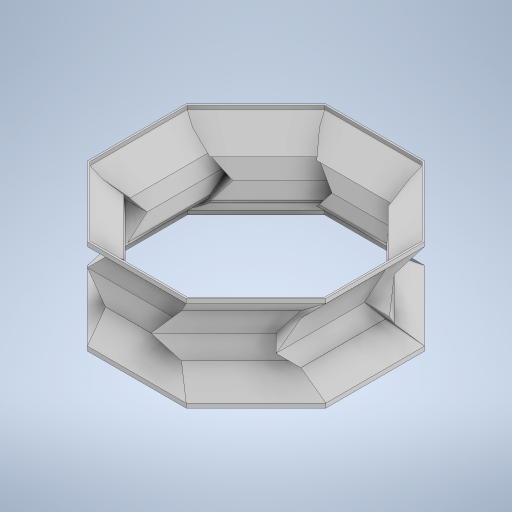
# Autodesk Inventor part: OV-PAM_new_shape
Saved by Autodesk Inventor 2024 (Build 280153000, 153)
## iProperties
Created: 2023-06-16
Part Number: OV-PAM_new_shape
Material: 일반
Document SubType Name: Modeling
Designer: jsw
Density: 1 g/cm^3
Appearance: 기본값
Author: jsw
Autodesk Inventor part; units mm, degrees
sketch "스케치1" plane through (0, 0, 0) normal (0, 1, 0) x (-1, 0, 0)
  line L0 (-32.5919, 13.5) -> (-13.5, 32.5919)
  line L1 (-13.5, 32.5919) -> (13.5, 32.5919)
  line L2 (13.5, 32.5919) -> (32.5919, 13.5)
  line L3 (32.5919, 13.5) -> (32.5919, -13.5)
  line L4 (32.5919, -13.5) -> (13.5, -32.5919)
  line L5 (13.5, -32.5919) -> (-13.5, -32.5919)
  line L6 (-13.5, -32.5919) -> (-32.5919, -13.5)
  line L7 (-32.5919, -13.5) -> (-32.5919, 13.5)
  line L8 (-13.7485, 33.1919) -> (13.7485, 33.1919)
  line L9 (13.7485, 33.1919) -> (33.1919, 13.7485)
  line L10 (33.1919, 13.7485) -> (33.1919, -13.7485)
  line L11 (33.1919, -13.7485) -> (13.7485, -33.1919)
  line L12 (13.7485, -33.1919) -> (-13.7485, -33.1919)
  line L13 (-13.7485, -33.1919) -> (-33.1919, -13.7485)
  line L14 (-33.1919, -13.7485) -> (-33.1919, 13.7485)
  line L15 (-33.1919, 13.7485) -> (-13.7485, 33.1919)
  point P0 (0, 0)
  point P1 (0, 0)
  point P2 (0, 0)
  dimension "d0" = 27
  dimension "d2" = 0.6
  constraints: 32 end point, 2 coincident, 2 horizontal, 34 other
  measures "d0" distance of L0.end L1.end
  measures "d2" distance between parallel lines of L10 L3
extrude "돌출2" add sketch "스케치1" along normal blind 12 contours L0 L1 L2 L3 L4 L5 L6 L7 | L8 L9 L10 L11 L12 L13 L14 L15
ref_plane "작업 평면2" through (33.1919, 0, 13.7485) normal (-0.8660254, -0.5, 0) x (0, 0, -1)
sketch "스케치3" plane through (33.1919, 0, 13.7485) normal (1, 0, 0) x (0, 0, -1)
  line L0 (0, 0) -> (0, 12) projected
  line L1 (0, 12) -> (27.4971, 12) projected
  line L2 (0, 0) -> (27.4971, 0)
  line L3 (27.4971, 0) -> (27.4971, 12)
  line L4 (27.4971, 12) -> (0, 12)
  line L5 (0, 12) -> (0, 0)
  line L6 (0, 12) -> (-7.3047, 12)
  line L7 (-19.4434, 12) -> (0, 12) projected
  line L8 (0, 0) -> (-7.3047, 12)
  line L9 (27.4971, 12) -> (13.7485, 12)
  line L10 (17.4971, 12) -> (27.4971, 0)
  point P0 (13.7485, 0)
  point P1 (17.4971, 12)
  dimension "d17" = 121.33
  dimension "d53" = 10
  constraints: 16 end point, 5 midpoint, 2 parallel, 2 point on line, 1 horizontal, 1 perpendicular
  measures "d17" angle of L8 L2
  measures "d53" distance of L1.end L10.start
extrude "돌출4" cut sketch "스케치3" against normal up to surface contours L8 L6 L0 | L0 L1 L10 L2 surface through (33.1919, 0, 13.7485) normal (-0.8660254, -0.5, 0)
pattern_circular "원형 패턴1" count 8 over 360 about axis through (0, -10, 0) along (0, 1, 0) of "돌출4"
ref_plane "작업 평면8" through (33.1919, 0, 13.7485) normal (-1, 0, 0) x (0, 0, -1)
sketch "스케치15" plane through (33.1919, 0, 13.7485) normal (-1, 0, 0) x (0, 0, -1)
  line L0 (0, 0) -> (-19.4434, 0) projected
  line L1 (0, 0) -> (27.4971, 0) projected
  line L2 (0, 0) -> (27.4971, 0)
  line L3 (22.5981, -6) -> (-3.5355, -6)
  line L4 (0, 0) -> (-3.5355, -6)
  line L5 (-7.0711, -12) -> (0, 0) projected
  line L6 (27.4971, 0) -> (22.5981, -6)
  line L7 (27.4971, 0) -> (17.6991, -12) projected
  point P0 (13.7485, 0)
  constraints: 8 end point, 2 midpoint, 1 collinear, 1 horizontal, 1 parallel
ref_plane "작업 평면9" through (33.1919, 0, 13.7485) normal (0.7071068, 0.7071068, 0) x (0, 0, -1)
extrude "돌출12" cut sketch "스케치15" along normal up to surface surface through (33.1919, 0, 13.7485) normal (0.7071068, 0.7071068, 0)
ref_plane "작업 평면10" through (26.2637, 12, 1.8262) normal (0.9876883, 0.1564345, 0) x (0, 0, -1)
sketch "스케치16" plane through (33.1919, 0, 13.7485) normal (-1, 0, 0) x (0, 0, -1)
  line L0 (-2.1721, -12) -> (-7.0711, -12) projected
  line L1 (22.5981, -6) -> (17.6991, -12) projected
  line L2 (-7.0711, -12) -> (17.6991, -12)
  line L3 (17.6991, -12) -> (22.5981, -6)
  line L4 (-7.0711, -12) -> (-3.5355, -6) projected
  line L5 (22.5981, -6) -> (-3.5355, -6)
  line L6 (-3.5355, -6) -> (-7.0711, -12)
  point P0 (13.7485, 0)
  constraints: 8 end point, 2 collinear, 1 horizontal, 1 parallel
extrude "돌출13" cut sketch "스케치16" along normal up to surface surface through (26.2637, 12, 1.8262) normal (0.9876883, 0.1564345, 0)
pattern_circular "원형 패턴3" count 8 over 360 about axis through (0, -10, 0) along (0, 1, 0) of "돌출12", "돌출13"
sketch "스케치17" plane through (0, 0, 0) normal (0, -1, 0) x (1, 0, 0)
  line L0 (33.1919, 13.7485) -> (33.1919, -13.7485) projected
  line L1 (13.7485, 33.1919) -> (33.1919, 13.7485) projected
  line L2 (-13.7485, 33.1919) -> (13.7485, 33.1919) projected
  line L3 (-33.1919, 13.7485) -> (-13.7485, 33.1919) projected
  line L4 (-33.1919, -13.7485) -> (-33.1919, 13.7485) projected
  line L5 (-13.7485, -33.1919) -> (-33.1919, -13.7485) projected
  line L6 (13.7485, -33.1919) -> (-13.7485, -33.1919) projected
  line L7 (33.1919, -13.7485) -> (13.7485, -33.1919) projected
  point P0 (0, 0)
extrude "돌출14" add sketch "스케치17" along normal blind 1.2
mirror "미러9" about plane through (0, 12, 0) normal (0, 1, 0) of "돌출12", "돌출13", "원형 패턴3", "돌출14", "돌출2"
shell "쉘7" thickness 0.5 removed faces 2 at (4.5828, 25.2, -1.8983) at (4.5828, -1.2, -1.8983)
